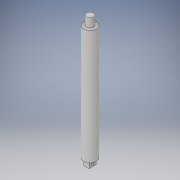
# Autodesk Inventor part: 9 inch Linear Actuator
Saved by Autodesk Inventor 2019 (Build 230136000, 136)
## iProperties
Created: 2018-11-15
Part Number: 9 inch Linear Actuator
Material: Generic
Document SubType Name: Modeling
Designer: Swapnil
Density: 1 g/cm^3
Appearance: Default
Author: Swapnil
Autodesk Inventor part; units mm, degrees
ref_plane "YZ Plane" through (0, 0, 0) normal (1, 0, 0) x (0, 1, 0)
ref_plane "XZ Plane" through (0, 0, 0) normal (0, 1, 0) x (-1, 0, 0)
ref_plane "XY Plane" through (0, 0, 0) normal (0, 0, 1) x (1, 0, 0)
sketch "Sketch1" plane through (0, 0, 0) normal (0, 1, 0) x (-1, 0, 0)
  circle A0 centre (0, 0) radius 18.034
  dimension "d0" = 36.068
  constraints: 1 centre point, 1 coincident
  measures "d0" diameter of A0
extrude "Extrusion1" add sketch "Sketch1" along normal blind 324.612
sketch "Sketch2" plane through (0, 324.612, 0) normal (0, 1, 0) x (1, 0, 0)
  circle A0 centre (0, 0) radius 9.525
  dimension "d3" = 19.05
  constraints: 1 centre point, 1 coincident
  measures "d3" diameter of A0
extrude "Extrusion2" add sketch "Sketch2" along normal blind 25.4
sketch "Sketch3" plane through (0, 0, 0) normal (0, -1, 0) x (1, 0, 0)
  line L0 (-7.62, -10.16) -> (7.62, -10.16)
  line L1 (7.62, -10.16) -> (7.62, 10.16)
  line L2 (7.62, 10.16) -> (-7.62, 10.16)
  line L3 (-7.62, 10.16) -> (-7.62, -10.16)
  line L4 (-7.62, -10.16) -> (7.62, 10.16) construction
  line L5 (7.62, -10.16) -> (-7.62, 10.16) construction
  point P0 (0, 0)
  dimension "d6" = 15.24
  dimension "d7" = 20.32
  constraints: 12 end point, 2 midpoint, 2 parallel, 1 horizontal, 1 perpendicular
  measures "d6" distance of L2.end L1.end
  measures "d7" distance of L1.end L0.end
extrude "Extrusion3" add sketch "Sketch3" along normal blind 18.288
sketch "Sketch4" plane through (7.62, 0, 10.16) normal (1, 0, 0) x (0, 0, -1)
  line L0 (0, 0) -> (20.32, 0) projected
  line L1 (20.32, 0) -> (20.32, -18.288) projected
  point P0 (10.16, 0)
  point P1 (10.16, -10.922)
  dimension "d10" = 10.922
  dimension "d11" = 10.16
  measures "d10" distance from line of L0 point (10.16, -10.922)
  measures "d11" distance from line of L1 point (10.16, -10.922)
hole "Hole1" at (7.62, -10.922, 0) direction (-1, 0, 0) diameter 6.35 end through all
sketch "Sketch5" plane through (7.62, 0, 10.16) normal (1, 0, 0) x (0, 0, -1)
  circle A0 centre (10.16, 340.614) radius 3.175
  line L0 (19.685, 350.012) -> (0.635, 350.012) projected
  point P0 (10.16, 0)
  dimension "d19" = 6.35
  dimension "d24" = 9.398
  constraints: 1 centre point
  measures "d19" diameter of A0
  measures "d24" distance from line of L0 A0.centre
extrude "Extrusion4" cut sketch "Sketch5" along normal mid plane 127
body "Solid1"
